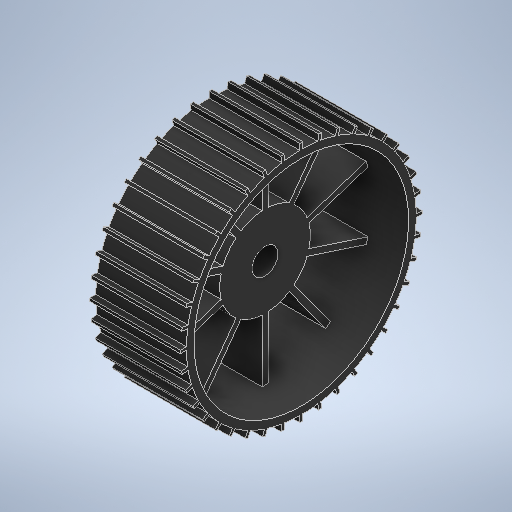
# Autodesk Inventor part: Roue libre
Saved by Autodesk Inventor 2026.2 (Build 302298010, 298A)
## iProperties
Created: 2026-04-01
Part Number: Roue libre
Material: Générique
Document SubType Name: Modeling
Designer: Genon
Density: 1 g/cm^3
Appearance: Caoutchouc - Noir
Author: Genon
Autodesk Inventor part; units mm, degrees
ref_plane "YZ Plane" through (0, 0, 0) normal (1, 0, 0) x (0, 1, 0)
ref_plane "XY Plane" through (0, 0, 0) normal (0, 0, 1) x (1, 0, 0)
sketch "Esquisse1" plane through (0, 0, 0) normal (0, 0, 1) x (1, 0, 0)
  line L0 (0, 0) -> (0, 15)
  line L1 (0, 15) -> (18, 15)
  line L2 (18, 15) -> (18, 0)
  line L3 (18, 0) -> (0, 0)
  line L4 (0, 0) -> (0, 38)
  line L5 (0, 38) -> (30, 38)
  line L6 (30, 38) -> (30, 35.5)
  line L7 (30, 35.5) -> (0, 35.5)
  dimension "d0" = 15
  dimension "d1" = 18
  dimension "d2" = 38
  dimension "d3" = 30
  dimension "d4" = 2.5
  constraints: 16 end point, 6 perpendicular, 2 point on line, 1 vertical
  measures "d0" distance of L0.start L0.end
  measures "d1" distance of L0.end L1.end
  measures "d2" distance of L0.start L4.end
  measures "d3" distance of L4.end L5.end
  measures "d4" distance of L5.end L6.end
revolve "Révolution1" add sketch "Esquisse1" angle 360 about axis through (18, 0, 0) along (-1, 0, 0)
ref_plane "Plan de construction1" through (0, 8, 0) normal (0, 1, 0) x (-1, 0, 0)
sketch "Esquisse2" plane through (0, 8, 0) normal (0, 1, 0) x (-1, 0, 0)
  line L0 (0, 0) -> (0, -1)
  line L1 (0, -38) -> (0, 38) projected
  line L2 (0, -1) -> (-18, -1)
  line L3 (-18, -1) -> (-18, 1)
  line L4 (-18, 1) -> (0, 1)
  line L5 (0, 0) -> (0, 1)
  dimension "d7" = 1
  dimension "d8" = 18
  dimension "d9" = 2
  constraints: 10 end point, 3 perpendicular, 2 point on line, 1 collinear
  measures "d7" distance of L0.start L0.end
  measures "d8" distance of L0.end L2.end
  measures "d9" distance of L2.end L3.end
extrude "Extrusion1" add sketch "Esquisse2" along normal up to surface round surface about axis through (15, 0, 0) along (-1, 0, 0) radius 38 far side no
sketch "Esquisse4" plane through (30, 0, 0) normal (1, 0, 0) x (0, 0, -1)
  circle A0 centre (0, 0) radius 38 projected
  circle A1 centre (0, 0) radius 38 projected
  line L0 (0, 38) -> (0, 40)
  line L1 (0, 40) -> (0.5, 40)
  line L2 (0.5, 40) -> (0.5, 37.9967)
  line L3 (0, 40) -> (-0.5, 40)
  line L4 (-0.5, 40) -> (-0.5, 37.9967)
  dimension "d15" = 2
  dimension "d16" = 0.5
  dimension "d17" = 0.5
  constraints: 10 end point, 3 perpendicular, 3 point on circle, 1 point on line, 1 vertical
  measures "d15" distance of L0.start L0.end
  measures "d16" distance of L0.end L1.end
  measures "d17" distance of L0.end L3.end
extrude "Extrusion2" add sketch "Esquisse4" against normal up to surface (30 mm away) contours A0 L0 L1 L2 | L4 L3 L0 A0
pattern_circular "Réseau circulaire1" count 40 over 360 about axis through (9, 0, 0) along (-1, 0, 0) of "Extrusion2"
pattern_circular "Réseau circulaire2" count 10 over 360 about axis through (9, 0, 0) along (-1, 0, 0) of "Extrusion1"
sketch "Esquisse5" plane through (0, 0, 0) normal (-1, 0, 0) x (0, -0.5224986, 0.8526402)
  circle A0 centre (0, 0) radius 11
  dimension "d26" = 22
  constraints: 1 centre point, 1 coincident
  measures "d26" diameter of A0
extrude "Extrusion3" cut sketch "Esquisse5" against normal blind 9
sketch "Esquisse6" plane through (9, 0, 0) normal (-1, 0, 0) x (0, 0, 1)
  circle A0 centre (0, 0) radius 7.5
  circle A1 centre (0, 0) radius 11 projected
  dimension "d30" = 15
  constraints: 1 centre point, 1 coincident
  measures "d30" diameter of A0
extrude "Extrusion4" add sketch "Esquisse6" along normal blind 1
sketch "Esquisse7" plane through (9, 0, 0) normal (-1, 0, 0) x (0, 0, 1)
  circle A0 centre (0, 0) radius 7.5 projected
  circle A1 centre (0, 0) radius 4.25
  dimension "d33" = 8.5
  constraints: 1 centre point, 1 coincident
  measures "d33" diameter of A1
extrude "Extrusion5" cut sketch "Esquisse7" against normal through all contours A1
